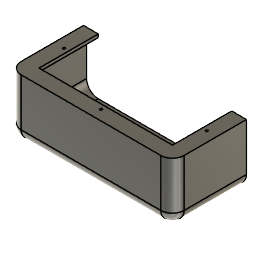
DropperBox (Autodesk Fusion 360 design; units mm, degrees)
Autodesk Fusion 360 part; units mm, degrees
sketch "Sketch1" plane through (0, 0, 0) normal (0, 0, 1) x (1, 0, 0)
  line L0 (0, 0) -> (171.45, 0)
  line L1 (171.45, 0) -> (171.45, 76.2)
  line L2 (171.45, 76.2) -> (0, 76.2)
  line L3 (0, 76.2) -> (0, 0)
  line L4 (-19.05, -19.05) -> (190.5, -19.05)
  line L5 (190.5, -19.05) -> (190.5, 95.25)
  line L6 (190.5, 95.25) -> (-19.05, 95.25)
  line L7 (-19.05, 95.25) -> (-19.05, -19.05)
  line L8 (0, 76.2) -> (-19.05, 76.2)
  line L9 (-19.05, 76.2) -> (171.45, 76.2)
  line L10 (171.45, 76.2) -> (190.5, 76.2)
  line L11 (186.5, 91.25) -> (-15.05, 91.25)
  line L12 (-15.05, 91.25) -> (-15.05, -15.05)
  line L13 (-15.05, -15.05) -> (186.5, -15.05)
  line L14 (186.5, -15.05) -> (186.5, 91.25)
  line L15 (0, 38.1) -> (-6, 38.1) construction
  line L16 (171.45, 38.1) -> (177.45, 38.1) construction
  circle A0 centre (-6, 38.1) radius 1.5
  circle A1 centre (177.45, 38.1) radius 1.5
  line L17 (85.725, 0) -> (85.725, -6) construction
  circle A2 centre (85.725, -6) radius 1.5
  dimension "d1" = 171.45
  dimension "d2" = 76.2
  dimension "d3" = 19.05
  dimension "d4" = -4
  dimension "d15" = 6
  dimension "d16" = 6
  dimension "d17" = 3
  dimension "d18" = 3
  dimension "d19" = 6
  dimension "d20" = 3
  constraint horizontal L0
  constraint vertical L1
  constraint horizontal L2
  constraint vertical L3
  constraint coincident L0.start L3.end
  constraint coincident L7 L8.end
  constraint perpendicular L7 L8
  constraint perpendicular L1 L10
  constraint coincident L5 L10.end
  constraint midpoint L3 L15.start
  constraint perpendicular L3 L15
  constraint midpoint L1 L16.start
  constraint perpendicular L1 L16
  constraint coincident L15.end A0.centre
  constraint coincident L16.end A1.centre
  constraint midpoint L0 L17.start
  constraint perpendicular L0 L17
  constraint coincident L17.end A2.centre
  measures "d1" distance of L0.start L0.end
  measures "d2" distance of L0.start L2.end
  measures "d15" distance of L15.start L15.end
  measures "d16" distance of L16.start L16.end
  measures "d17" diameter of A0
  measures "d18" diameter of A1
  measures "d19" distance of L17.start L17.end
  measures "d20" diameter of A2
extrude "Extrude1" add sketch "Sketch1" against normal blind 76.2 contours L0 L1 L3 L8 L9 L10 L12 L13 L14 | L4 L5 L7 L8 L9 L10 L12 L13 L14 | A0 | A1 | A2
extrude "Extrude2" add sketch "Sketch1" along normal blind 4 from surface at -76.2 contours L0 L1 L2 L3 L9 | L0 L1 L3 L8 L9 L10 L12 L13 L14 | L4 L5 L7 L8 L9 L10 L12 L13 L14 | A0 | A1 | A2
extrude "Extrude3" cut sketch "Sketch1" along normal blind 68 from surface at -72.2 contours L0 L1 L3 L8 L9 L10 L12 L13 L14 | A0 | A1 | A2
fillet "Fillet1" radius 15 13 edges at (-15.05, 30.575, -72.2) (85.725, -15.05, -72.2) (-15.05, -15.05, -38.2) (-15.05, 30.575, -4.2) (85.725, -15.05, -4.2) (186.5, 30.575, -4.2) (186.5, 30.575, -72.2) (186.5, -15.05, -38.2) (-19.05, -19.05, -38.1) (-19.05, 28.575, -76.2) (85.725, -19.05, -76.2) (190.5, 28.575, -76.2) (190.5, -19.05, -38.1)
extrude "Extrude4" cut sketch "Sketch1" against normal blind 20 contours A0 | A1 | A2
